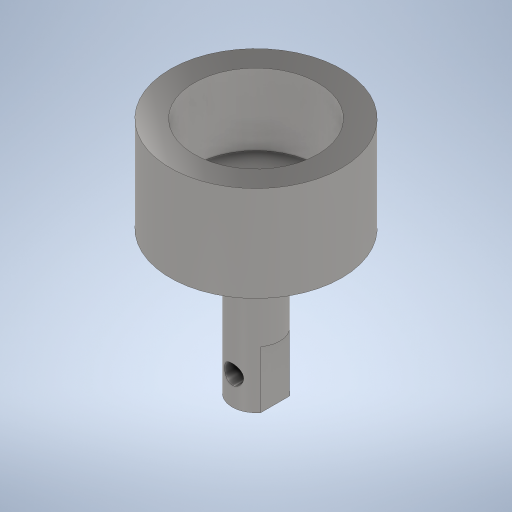
# Autodesk Inventor part: shellerAdapter
Saved by Autodesk Inventor 2024.2 (Build 282272000, 272)
## iProperties
Created: 2024-05-29
Part Number: shellerAdapter
Material: Stainless Steel, Austenitic
Document SubType Name: Modeling
Designer: user
Density: 8 g/cm^3
Appearance: Semi-Polished
Author: user
Autodesk Inventor part; units mm, degrees
ref_plane "YZ Plane" through (0, 0, 0) normal (1, 0, 0) x (0, 1, 0)
ref_plane "XZ Plane" through (0, 0, 0) normal (0, 1, 0) x (-1, 0, 0)
ref_plane "XY Plane" through (0, 0, 0) normal (0, 0, 1) x (1, 0, 0)
sketch "Sketch1" plane through (0, 0, 0) normal (0, 0, 1) x (1, 0, 0)
  line L0 (0, 0) -> (0, 50)
  line L1 (0, 50) -> (18, 50)
  line L2 (18, 50) -> (18, 30)
  line L3 (18, 30) -> (5, 30)
  line L4 (5, 30) -> (5, 0)
  line L5 (5, 0) -> (0, 0)
  dimension "d0" = 50
  dimension "d1" = 18
  dimension "d2" = 20
  dimension "d3" = 13
  constraints: 12 end point, 5 perpendicular, 1 vertical
  measures "d0" distance of L0.start L0.end
  measures "d1" distance of L0.end L1.end
  measures "d2" distance of L1.end L2.end
  measures "d3" distance of L2.end L3.end
revolve "Revolution1" add sketch "Sketch1" angle 360 about axis through (0, 0, 0) along (0, 1, 0)
sketch "Sketch2" plane through (0, 50, 0) normal (0, 1, 0) x (1, 0, 0)
  circle A0 centre (0, 0) radius 18 projected
  circle A1 centre (0, 0) radius 13
  dimension "d5" = 5
  constraints: 1 centre point
  measures "d5" radial gap between concentric circles of A0 A1
extrude "Extrusion1" cut sketch "Sketch2" against normal blind 15 contours A1
sketch "Sketch3" plane through (0, 0, 0) normal (0, 0, 1) x (1, 0, 0)
  line L0 (5, 0) -> (-5, 0) projected
  line L1 (5, 12) -> (-5, 12)
  line L2 (5, 12) -> (4, 12)
  line L3 (4, 12) -> (4, 0)
  line L4 (4, 0) -> (5, 0)
  line L5 (5, 0) -> (5, 12)
  point P0 (0, 0)
  dimension "d8" = 12
  constraints: 10 end point, 3 parallel, 1 horizontal, 1 perpendicular, 1 point on line
  measures "d8" distance between parallel lines of L0 L1
extrude "Extrusion2" cut sketch "Sketch3" along normal through all both and the other way through all
sketch "Sketch4" plane through (0, 0, 0) normal (0, 0, 1) x (1, 0, 0)
  line L0 (4, 0) -> (-5, 0) projected
  circle A0 centre (0, 6) radius 2
  point P0 (0, 0)
  dimension "d11" = 6
  dimension "d12" = 4
  constraints: 1 centre point, 1 coincident
  measures "d11" distance from line of L0 point (0, 6)
  measures "d12" diameter of A0
extrude "Extrusion3" cut sketch "Sketch4" along normal through all both and the other way through all
body "Solid1"
